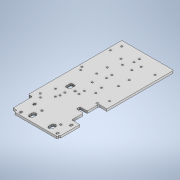
# Autodesk Inventor part: Top Divider
Saved by Autodesk Inventor 2021 (Build 250183000, 183)
## iProperties
Created: 2020-07-14
Part Number: Top Divider
Material: Generic
Document SubType Name: Modeling
Designer: jgray
Density: 1 g/cm^3
Appearance: Default
Author: jgray
Autodesk Inventor part; units mm, degrees
ref_plane "YZ Plane" through (0, 0, 0) normal (1, 0, 0) x (0, 1, 0)
ref_plane "XZ Plane" through (0, 0, 0) normal (0, 1, 0) x (-1, 0, 0)
ref_plane "XY Plane" through (0, 0, 0) normal (0, 0, 1) x (1, 0, 0)
sketch "Sketch1" plane through (0, 0, 0) normal (0, 1, 0) x (-1, 0, 0)
  line L0 (0, 0) -> (107.2, 0)
  line L1 (116.2, -52) -> (116.2, -262)
  line L2 (116.2, -262) -> (0, -262)
  line L3 (0, -262) -> (0, 0)
  line L4 (107.2, 0) -> (107.2, -52)
  line L5 (107.2, -52) -> (116.2, -52)
  dimension "d4" = 9
  dimension "d5" = 107.2
  dimension "d6" = 210
  dimension "d7" = 262
  constraints: 12 end point, 2 parallel, 1 horizontal, 1 perpendicular
  measures "d4" distance of L4.end L1.start
  measures "d5" distance of L0.start L0.end
  measures "d6" distance of L1.start L1.end
  measures "d7" distance of L2.end L0.start
extrude "Extrusion1" add sketch "Sketch1" along normal blind 5
fillet "Fillet1" radius 2 3 edges at (-116.2, 2.5, -52) (-107.2, 2.5, -52) (0, 2.5, -262)
sketch "Sketch2" plane through (0, 5, 0) normal (0, 1, 0) x (1, 0, 0)
  line L0 (-12, -58.0921) -> (-12, 320.7627) construction
  line L1 (-43, -58.0921) -> (-43, 320.7627) construction
  line L2 (-149.1257, 232) -> (35.6079, 232) construction
  line L3 (-154.8253, 130) -> (27.8967, 130) construction
  line L4 (-114.2, 52) -> (-109.2, 52) construction
  line L5 (0, 0) -> (0, 260) projected
  line L6 (-2, 262) -> (-116.2, 262) projected
  point P0 (-43, 130)
  point P1 (-12, 130)
  point P2 (-43, 232)
  point P3 (-12, 232)
  point P4 (0, 2)
  point P5 (-114.2, 262)
  dimension "d20" = 12
  dimension "d21" = 31
  dimension "d43" = 30
  dimension "d44" = 102
  constraints: 8 end point, 8 point on line, 2 horizontal, 2 vertical
  measures "d20" distance between parallel lines of L5 L0
  measures "d21" distance between parallel lines of L0 L1
  measures "d43" distance from line of point (-12, 232) L6
  measures "d44" distance of point (-12, 130) point (-12, 232)
hole "Hole1" at (-43, 5, -130) at (-12, 5, -130) at (-43, 5, -232) at (-12, 5, -232) direction (0, -1, 0) diameter 3.8 end through all
sketch "Sketch3" plane through (0, 5, 0) normal (0, 1, 0) x (1, 0, 0)
  line L0 (0, 0) -> (0, 260) projected
  line L1 (-8.0112, 9.3) -> (-90.01, 8.86) construction
  line L2 (-90.01, 8.86) -> (-90.1763, 39.8596) construction
  line L3 (-90.1763, 39.8596) -> (-8.1775, 40.2996) construction
  line L4 (-8.1775, 40.2996) -> (-8.0112, 9.3) construction
  line L5 (-8.0112, 9.3) -> (-90.1763, 39.8596) construction
  line L6 (-90.01, 8.86) -> (-8.1775, 40.2996) construction
  line L7 (-107.2, 0) -> (0, 0) projected
  line L8 (-90.0046, 7.86) -> (-90.0154, 9.86) construction
  line L9 (-87.6047, 7.8729) -> (-87.6154, 9.8729)
  line L10 (-92.4153, 9.8471) -> (-92.4046, 7.8471)
  arc A0 (-92.4046, 7.8471) -> (-87.6047, 7.8729) centre (-90.0046, 7.86) ccw
  arc A1 (-87.6154, 9.8729) -> (-92.4153, 9.8471) centre (-90.0154, 9.86) ccw
  line L11 (-90.171, 38.8596) -> (-90.1817, 40.8595) construction
  line L12 (-87.771, 38.8724) -> (-87.7817, 40.8724)
  line L13 (-92.5817, 40.8467) -> (-92.5709, 38.8467)
  arc A2 (-92.5709, 38.8467) -> (-87.771, 38.8724) centre (-90.171, 38.8596) ccw
  arc A3 (-87.7817, 40.8724) -> (-92.5817, 40.8467) centre (-90.1817, 40.8595) ccw
  line L14 (-8.1722, 39.2996) -> (-8.1829, 41.2995) construction
  line L15 (-5.7722, 39.3124) -> (-5.7829, 41.3124)
  line L16 (-10.5829, 41.2867) -> (-10.5721, 39.2867)
  arc A4 (-10.5721, 39.2867) -> (-5.7722, 39.3124) centre (-8.1722, 39.2996) ccw
  arc A5 (-5.7829, 41.3124) -> (-10.5829, 41.2867) centre (-8.1829, 41.2995) ccw
  line L17 (-8.0058, 8.3) -> (-8.0165, 10.3) construction
  line L18 (-5.6058, 8.3129) -> (-5.6166, 10.3129)
  line L19 (-10.4165, 10.2871) -> (-10.4058, 8.2871)
  arc A6 (-10.4058, 8.2871) -> (-5.6058, 8.3129) centre (-8.0058, 8.3) ccw
  arc A7 (-5.6166, 10.3129) -> (-10.4165, 10.2871) centre (-8.0165, 10.3) ccw
  point P0 (-90.1763, 39.8596)
  point P1 (0, 2)
  point P2 (-49.0938, 24.5798)
  point P3 (-105.2, 0)
  point P4 (-2, 0)
  point P5 (-90.1763, 39.8596)
  point P6 (-90.1763, 39.8596)
  point P7 (-8.1775, 40.2996)
  point P8 (-8.1775, 40.2996)
  point P9 (-8.0112, 9.3)
  point P10 (-8.0112, 9.3)
  dimension "d24" = 82
  dimension "d25" = 31
  dimension "d26" = 8.86
  dimension "d27" = 90.01
  dimension "d28" = 9.3
  dimension "d29" = 40.2996
  dimension "d30" = 39.8595
  dimension "d31" = 1
  dimension "d32" = 4.8
  dimension "d33" = 1
  dimension "d34" = 4.8
  dimension "d35" = 1
  dimension "d36" = 4.8
  dimension "d37" = 1
  dimension "d38" = 4.8
  dimension "d41" = 81.9988
  dimension "d42" = 0.1663
  constraints: 44 end point, 16 point on circle, 16 tangent, 8 centre point, 8 parallel, 7 coincident, 7 point on line, 6 midpoint, 1 perpendicular
  measures "d24" distance of L1.start L1.end
  measures "d25" distance of L1.end L2.end
  measures "d26" distance from line of L7 L1.end
  measures "d27" distance from line of L0 L1.end
  measures "d28" distance from line of L7 L1.start
  measures "d29" distance from line of L3.end L7
  measures "d30" distance from line of L7 L2.end
  measures "d31" distance of L1.end L8.end
  measures "d32" diameter of A1
  measures "d33" distance of point (-90.176, 39.86) L11.end
  measures "d34" diameter of A3
  measures "d35" distance of point (-8.178, 40.3) L14.end
  measures "d36" diameter of A5
  measures "d37" distance of point (-8.011, 9.3) L17.end
  measures "d38" diameter of A7
  measures "d41" horizontal distance of L2.end L3.end
  measures "d42" horizontal distance of L3.end L1.start
extrude "Extrusion2" cut sketch "Sketch3" against normal through all
sketch "Sketch4" plane through (0, 5, 0) normal (0, 1, 0) x (1, 0, 0)
  line L0 (0, 0) -> (0, 260) projected
  line L1 (0, 112) -> (-18, 112)
  line L2 (-18, 112) -> (-18, 51)
  line L3 (-18, 51) -> (0, 51)
  line L4 (0, 51) -> (0, 112)
  line L5 (-2, 262) -> (-116.2, 262) projected
  point P0 (0, 2)
  point P1 (-114.2, 262)
  point P2 (0, 51)
  dimension "d45" = 61
  dimension "d46" = 150
  dimension "d47" = 18
  constraints: 8 end point, 2 parallel, 1 horizontal, 1 perpendicular, 1 point on line
  measures "d45" distance from line of L2.end L1
  measures "d46" distance between parallel lines of L5 L1
  measures "d47" distance between parallel lines of L0 L2
extrude "Extrusion3" cut sketch "Sketch4" against normal through all
fillet "Fillet2" radius 2 2 edges at (-18, 2.5, -112) (-18, 2.5, -51)
sketch "Sketch5" plane through (0, 5, 0) normal (0, 1, 0) x (1, 0, 0)
  line L0 (-190.0868, 16.45) -> (100.3829, 16.45) construction
  line L1 (-71.05, 85.7374) -> (-71.05, -34.478) construction
  line L2 (-116.2, 262) -> (-116.2, 54) construction
  line L3 (-27.05, 83.5) -> (-27.05, -34.478) construction
  line L4 (-107.2, 0) -> (0, 0) construction
  line L5 (-107.2, 50) -> (-107.2, 0) construction
  line L6 (-27.05, 13.45) -> (-27.05, 19.45)
  line L7 (-22.3, 13.45) -> (-22.3, 19.45)
  line L8 (-31.8, 19.45) -> (-31.8, 13.45)
  arc A0 (-31.8, 13.45) -> (-22.3, 13.45) centre (-27.05, 13.45) ccw
  arc A1 (-22.3, 19.45) -> (-31.8, 19.45) centre (-27.05, 19.45) ccw
  line L9 (-71.05, 13.45) -> (-71.05, 19.45)
  line L10 (-66.3, 13.45) -> (-66.3, 19.45)
  line L11 (-75.8, 19.45) -> (-75.8, 13.45)
  arc A2 (-75.8, 13.45) -> (-66.3, 13.45) centre (-71.05, 13.45) ccw
  arc A3 (-66.3, 19.45) -> (-75.8, 19.45) centre (-71.05, 19.45) ccw
  point P0 (-116.2, 260)
  point P1 (-105.2, 0)
  point P2 (-2, 0)
  point P3 (-107.2, 2)
  point P4 (-27.05, 16.45)
  point P5 (-71.05, 16.45)
  dimension "d51" = 16.45
  dimension "d52" = 36.15
  dimension "d53" = 80.15
  dimension "d54" = 3
  dimension "d55" = 9.5
  dimension "d56" = 3
  dimension "d57" = 9.5
  constraints: 22 end point, 8 point on circle, 8 tangent, 5 point on line, 4 centre point, 3 parallel, 2 midpoint, 1 horizontal, 1 vertical
  measures "d51" distance between parallel lines of L0 L4
  measures "d52" distance between parallel lines of L1 L5
  measures "d53" distance between parallel lines of L3 L5
  measures "d54" distance of point (-27.05, 16.45) L6.end
  measures "d55" diameter of A1
  measures "d56" distance of point (-71.05, 16.45) L9.end
  measures "d57" diameter of A3
extrude "Extrusion4" cut sketch "Sketch5" against normal blind 10
sketch "Sketch6" plane through (0, 5, 0) normal (0, 1, 0) x (1, 0, 0)
  line L0 (-78.7, 111.8556) -> (-78.7, -42.3162) construction
  line L1 (-135.3054, 85.54) -> (-37.9202, 85.54) construction
  line L2 (-134.0207, 96.54) -> (-37.9202, 96.54) construction
  line L3 (-116.2, 262) -> (-116.2, 54) construction
  line L4 (-107.2, 0) -> (0, 0) construction
  point P0 (-116.2, 260)
  point P1 (-105.2, 0)
  point P2 (-2, 0)
  point P3 (-78.7, 96.54)
  point P4 (-78.7, 85.54)
  dimension "d60" = 37.5
  dimension "d61" = 85.54
  dimension "d62" = 96.54
  constraints: 6 end point, 4 point on line, 2 horizontal, 1 vertical
  measures "d60" distance between parallel lines of L0 L3
  measures "d61" distance between parallel lines of L4 L1
  measures "d62" distance between parallel lines of L2 L4
hole "Hole2" at (-78.7, 5, -96.54) at (-78.7, 5, -85.54) direction (0, -1, 0) diameter 3.8 end through all
sketch "Sketch7" plane through (-107.2, 0, 0) normal (0, 0, 1) x (1, 0, 0)
  line L0 (0, 0) -> (107.2, 0) projected
  line L1 (107.2, 0) -> (107.2, 5) projected
  line L2 (0, 5) -> (107.2, 5) projected
  line L3 (0, 0) -> (0, 5) projected
  line L4 (0, 0) -> (107.2, 0)
  line L5 (107.2, 0) -> (107.2, 5)
  line L6 (107.2, 5) -> (0, 5)
  line L7 (0, 5) -> (0, 0)
  constraints: 8 end point, 2 parallel, 1 horizontal, 1 perpendicular
extrude "Extrusion5" cut sketch "Sketch7" against normal blind 2.5
sketch "Sketch8" plane through (0, 5, 0) normal (0, 1, 0) x (1, 0, 0)
  line L0 (-107.2, 2.5) -> (0, 2.5) projected
  line L1 (0, 112) -> (0, 51) projected
  point P0 (0, 0)
  point P1 (-21.12, 29.5)
  point P2 (-69.429, 35.592)
  point P3 (-69.82, 110.52)
  point P4 (-21.56, 112.05)
  point P5 (-103.2, 2.5)
  point P6 (-4, 2.5)
  point P7 (0, 6.5)
  dimension "d74" = 27
  dimension "d75" = 21.12
  dimension "d76" = 33.092
  dimension "d77" = 69.429
  dimension "d80" = 109.55
  dimension "d81" = 108.02
  dimension "d82" = 21.56
  dimension "d83" = 69.82
  measures "d74" distance from line of point (-21.12, 29.5) L0
  measures "d75" distance from line of point (-21.12, 29.5) L1
  measures "d76" distance from line of L0 point (-69.429, 35.592)
  measures "d77" distance from line of L1 point (-69.429, 35.592)
  measures "d80" distance from line of L0 point (-21.56, 112.05)
  measures "d81" distance from line of point (-69.82, 110.52) L0
  measures "d82" distance from line of L1 point (-21.56, 112.05)
  measures "d83" distance from line of L1 point (-69.82, 110.52)
hole "Hole3" at (-21.12, 5, -29.5) at (-69.429, 5, -35.592) at (-69.82, 5, -110.52) at (-21.56, 5, -112.05) direction (0, -1, 0) diameter 4.5 end through all
sketch "Sketch10" plane through (0, 5, 0) normal (0, 1, 0) x (1, 0, 0)
  line L0 (-60, 244.888) -> (-60, 121.612) construction
  line L1 (0, 112) -> (0, 260) construction
  line L2 (-2, 262) -> (-116.2, 262) construction
  point P0 (0, 0)
  point P1 (-60, 245)
  point P2 (-60, 233)
  point P3 (-114.2, 262)
  point P4 (-60, 183.25)
  point P5 (-60, 171.25)
  dimension "d102" = 60
  dimension "d103" = 17
  dimension "d104" = 12
  dimension "d105" = 61.75
  dimension "d106" = 61.75
  constraints: 3 point on line, 2 end point, 1 midpoint, 1 vertical
  measures "d102" distance between parallel lines of L1 L0
  measures "d103" distance from line of L2 point (-60, 245)
  measures "d104" distance of point (-60, 233) point (-60, 245)
  measures "d105" distance of point (-60, 183.25) point (-60, 245)
  measures "d106" distance of point (-60, 233) point (-60, 171.25)
hole "Hole5" at (-60, 5, -245) at (-60, 5, -233) at (-60, 5, -183.25) at (-60, 5, -171.25) direction (0, -1, 0) diameter 3.8 end through all
sketch "Sketch11" plane through (0, 5, 0) normal (0, 1, 0) x (1, 0, 0)
  line L0 (-179.761, 133.5) -> (45.4036, 133.5) construction
  line L1 (-2, 262) -> (-116.2, 262) construction
  line L2 (-60, 306.7904) -> (-60, 56.1772) construction
  line L3 (0, 112) -> (0, 260) construction
  point P0 (0, 0)
  point P1 (-114.2, 262)
  point P2 (-60, 121.5)
  point P3 (-60, 109.5)
  dimension "d114" = 128.5
  dimension "d115" = 60
  dimension "d116" = 12
  dimension "d117" = 12
  constraints: 4 end point, 2 point on line, 1 horizontal, 1 vertical
  measures "d114" distance between parallel lines of L0 L1
  measures "d115" distance between parallel lines of L3 L2
  measures "d116" distance from line of L0 point (-60, 121.5)
  measures "d117" distance of point (-60, 109.5) point (-60, 121.5)
hole "Hole6" at (-60, 5, -121.5) at (-60, 5, -109.5) direction (0, -1, 0) diameter 3.8 end through all
sketch "Sketch12" plane through (0, 5, 0) normal (0, 1, 0) x (1, 0, 0)
  line L0 (-109.7, 283.3121) -> (-109.7, 62.2956) construction
  line L1 (-116.2, 262) -> (-116.2, 54) projected
  line L2 (-2, 262) -> (-116.2, 262) projected
  point P0 (0, 0)
  point P1 (-109.7, 229.75)
  point P2 (-109.7, 165.75)
  dimension "d125" = 6.5
  dimension "d126" = 32.25
  dimension "d127" = 64
  constraints: 2 end point, 2 point on line, 1 vertical
  measures "d125" distance between parallel lines of L0 L1
  measures "d126" distance from line of point (-109.7, 229.75) L2
  measures "d127" distance of point (-109.7, 165.75) point (-109.7, 229.75)
hole "Hole7" at (-109.7, 5, -229.75) at (-109.7, 5, -165.75) direction (0, -1, 0) diameter 3.8 end through all
sketch "Sketch13" plane through (0, 5, 0) normal (0, 1, 0) x (1, 0, 0)
  line L0 (-96.7, 282.6166) -> (-96.7, 46.4952) construction
  line L1 (-116.2, 262) -> (-116.2, 54) projected
  line L2 (-2, 262) -> (-116.2, 262) projected
  point P0 (0, 0)
  point P1 (-96.7, 93.5)
  point P2 (-96.7, 59.5)
  dimension "d135" = 19.5
  dimension "d136" = 168.5
  dimension "d137" = 34
  constraints: 2 end point, 2 point on line, 1 vertical
  measures "d135" distance between parallel lines of L0 L1
  measures "d136" distance from line of point (-96.7, 93.5) L2
  measures "d137" distance of point (-96.7, 93.5) point (-96.7, 59.5)
hole "Hole8" at (-96.7, 5, -93.5) at (-96.7, 5, -59.5) direction (0, -1, 0) diameter 3.8 end through all
sketch "Sketch14" plane through (0, 5, 0) normal (0, 1, 0) x (1, 0, 0)
  line L0 (-104.7, 331.3902) -> (-104.7, -52.1712) construction
  line L1 (-116.2, 262) -> (-116.2, 54) construction
  line L2 (-2, 262) -> (-116.2, 262) construction
  point P0 (0, 0)
  point P1 (-104.7, 67)
  point P2 (-104.7, 158)
  point P3 (-104.7, 250)
  dimension "d145" = 11.5
  dimension "d146" = 12
  dimension "d147" = 104
  dimension "d148" = 195
  constraints: 3 point on line, 2 end point, 1 vertical
  measures "d145" distance between parallel lines of L0 L1
  measures "d146" distance from line of point (-104.7, 250) L2
  measures "d147" distance from line of point (-104.7, 158) L2
  measures "d148" distance from line of point (-104.7, 67) L2
hole "Hole9" at (-104.7, 5, -67) at (-104.7, 5, -158) at (-104.7, 5, -250) direction (0, -1, 0) diameter 3.8 end through all
sketch "Sketch15" plane through (0, 5, 0) normal (0, 1, 0) x (1, 0, 0)
  line L0 (-90.2, 122) -> (-80.2, 122)
  line L1 (-80.2, 122) -> (-80.2, 108)
  line L2 (-80.2, 108) -> (-90.2, 108)
  line L3 (-90.2, 108) -> (-90.2, 122)
  line L4 (-116.2, 262) -> (-116.2, 54) projected
  line L5 (-2, 262) -> (-116.2, 262) projected
  point P0 (0, 0)
  dimension "d156" = 10
  dimension "d157" = 14
  dimension "d158" = 26
  dimension "d159" = 140
  constraints: 8 end point, 2 parallel, 1 horizontal, 1 perpendicular
  measures "d156" distance of L1.end L2.end
  measures "d157" distance of L0.end L1.end
  measures "d158" distance between parallel lines of L4 L3
  measures "d159" distance from line of L5 L0.start
extrude "Extrusion6" cut sketch "Sketch15" against normal through all
fillet "Fillet5" radius 2 4 edges at (-90.2, 2.5, -122) (-80.2, 2.5, -122) (-80.2, 2.5, -108) (-90.2, 2.5, -108)
sketch "Sketch16" plane through (0, 5, 0) normal (0, 1, 0) x (1, 0, 0)
  line L0 (-107.2, 50) -> (-107.2, 2.5) projected
  line L1 (-107.2, 2.5) -> (-98.2, 2.5)
  line L2 (-98.2, 2.5) -> (-98.2, 8.5)
  line L3 (-98.2, 8.5) -> (-107.2, 8.5)
  line L4 (-107.2, 8.5) -> (-107.2, 2.5)
  line L5 (-107.2, 2.5) -> (0, 2.5) projected
  line L6 (0, 2.5) -> (-2, 2.5)
  line L7 (-2, 2.5) -> (-2, 8.5)
  line L8 (-2, 8.5) -> (0, 8.5)
  line L9 (0, 8.5) -> (0, 2.5)
  point P0 (0, 0)
  dimension "d163" = 9
  dimension "d164" = 6
  dimension "d165" = 2
  dimension "d166" = 6
  constraints: 16 end point, 4 parallel, 2 horizontal, 2 perpendicular
  measures "d163" distance of L3.end L2.end
  measures "d164" distance of L2.end L1.end
  measures "d165" distance of L7.end L8.end
  measures "d166" distance of L6.end L7.end
extrude "Extrusion7" cut sketch "Sketch16" against normal through all
fillet "Fillet6" radius 2 4 edges at (-2, 2.5, -8.5) (-2, 2.5, -2.5) (-98.2, 2.5, -2.5) (-98.2, 2.5, -8.5)
sketch "Sketch17" plane through (0, 5, 0) normal (0, 1, 0) x (1, 0, 0)
  line L0 (-18, 53) -> (-18, 102)
  line L1 (-34, 85.5) -> (-18, 85.5)
  line L2 (-18, 85.5) -> (-18, 77.5)
  line L3 (-18, 77.5) -> (-34, 77.5)
  line L4 (-34, 77.5) -> (-34, 85.5)
  line L5 (-48.5608, 81.5) -> (-5.1169, 81.5) construction
  line L6 (-16, 112) -> (0, 112) projected
  line L7 (0, 8.5) -> (0, 51) projected
  point P0 (0, 0)
  point P1 (-18, 81.5)
  dimension "d170" = 8
  dimension "d171" = 30.5
  dimension "d172" = 34
  constraints: 12 end point, 2 horizontal, 2 midpoint, 2 parallel, 1 perpendicular, 1 point on line
  measures "d170" distance between parallel lines of L1 L3
  measures "d171" distance between parallel lines of L5 L6
  measures "d172" distance between parallel lines of L7 L4
extrude "Extrusion8" cut sketch "Sketch17" against normal through all
fillet "Fillet7" radius 2 4 edges at (-18, 2.5, -85.5) (-34, 2.5, -85.5) (-34, 2.5, -77.5) (-18, 2.5, -77.5)
sketch "Sketch18" plane through (0, 5, 0) normal (0, 1, 0) x (1, 0, 0)
  line L0 (-81.5, 293.9819) -> (-81.5, -46.0174) construction
  line L1 (0, 112) -> (0, 260) projected
  line L2 (-2, 262) -> (-116.2, 262) projected
  point P0 (0, 0)
  point P1 (-81.5, 225)
  point P2 (-81.5, 78)
  dimension "d176" = 81.5
  dimension "d177" = 37
  dimension "d178" = 147
  constraints: 2 end point, 2 point on line, 1 vertical
  measures "d176" distance between parallel lines of L1 L0
  measures "d177" distance from line of L2 point (-81.5, 225)
  measures "d178" distance of point (-81.5, 78) point (-81.5, 225)
hole "Hole10" at (-81.5, 5, -225) at (-81.5, 5, -78) direction (0, -1, 0) diameter 3.8 end through all
sketch "Sketch19" plane through (0, 5, 0) normal (0, 1, 0) x (1, 0, 0)
  line L0 (-77, 212) -> (-34, 212) construction
  line L1 (-34, 212) -> (-34, 150) construction
  line L2 (-34, 150) -> (-77, 150) construction
  line L3 (-77, 150) -> (-77, 212) construction
  line L4 (0, 112) -> (0, 260) construction
  line L5 (-31, 215) -> (-80, 215) construction
  line L6 (-80, 215) -> (-80, 147) construction
  line L7 (-80, 147) -> (-31, 147) construction
  line L8 (-31, 147) -> (-31, 215) construction
  line L9 (-2, 262) -> (-116.2, 262) projected
  point P0 (0, 0)
  point P1 (-47, 215)
  point P2 (-68, 215)
  point P3 (-80, 193)
  point P4 (-80, 169)
  point P5 (-68, 147)
  point P6 (-47, 147)
  point P7 (-31, 193)
  point P8 (-31, 169)
  dimension "d186" = 43
  dimension "d187" = 62
  dimension "d188" = 34
  dimension "d189" = 3
  dimension "d191" = 12
  dimension "d192" = 21
  dimension "d193" = 21
  dimension "d194" = 12
  dimension "d195" = 22
  dimension "d196" = 22
  dimension "d204" = 22
  dimension "d205" = 22
  dimension "d206" = 47
  constraints: 16 end point, 8 point on line, 4 parallel, 2 perpendicular, 1 horizontal, 3 other
  measures "d186" distance of L1.end L2.end
  measures "d187" distance of L0.end L1.end
  measures "d188" distance between parallel lines of L4 L1
  measures "d189" distance between parallel lines of L0 L5
  measures "d191" distance from line of point (-68, 215) L6
  measures "d192" distance of point (-47, 215) point (-68, 215)
  measures "d193" distance of point (-68, 147) point (-47, 147)
  measures "d194" distance of point (-68, 147) L6.end
  measures "d195" distance from line of point (-80, 193) L5
  measures "d196" distance from line of L7 point (-80, 169)
  measures "d204" distance of point (-31, 169) L7.end
  measures "d205" distance of point (-31, 193) L5.start
  measures "d206" distance from line of L9 L5.start
hole "Hole11" at (-47, 5, -215) at (-68, 5, -215) at (-80, 5, -193) at (-80, 5, -169) at (-68, 5, -147) at (-47, 5, -147) at (-31, 5, -193) at (-31, 5, -169) direction (0, -1, 0) diameter 3.8 end through all
equation "\"d32\" = d34"
equation "\"d36\" = d34"
equation "\"d38\" = d34"
equation "\"d106\" = d105"
body "Solid1"
